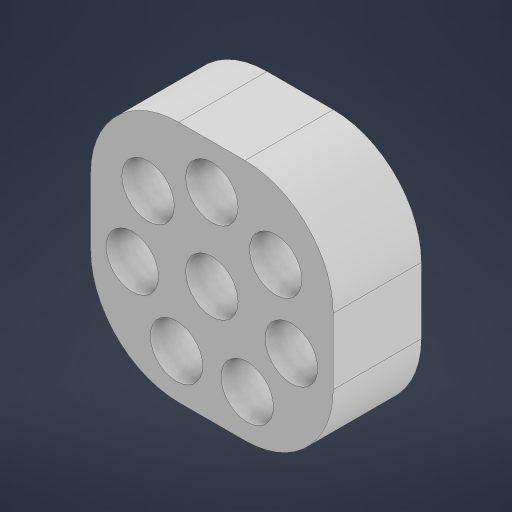
# Autodesk Inventor part: ShooterMount-1in
Saved by Autodesk Inventor 2023 (Build 270158000, 158)
## iProperties
Created: 2022-04-16
Part Number: ShooterMount-1in
Material: Generic
Document SubType Name: Modeling
Designer: timmy
Density: 1 g/cm^3
Appearance: Default
Author: timmy
Autodesk Inventor part; units mm, degrees
ref_plane "YZ Plane" through (0, 0, 0) normal (1, 0, 0) x (0, 1, 0)
sketch "Sketch1" plane through (0, 0, 0) normal (0, 0, 1) x (1, 0, 0)
  line L0 (0, 0) -> (279.4, 0)
  line L1 (279.4, 0) -> (279.4, 279.4)
  line L2 (279.4, 279.4) -> (0, 279.4)
  line L3 (0, 279.4) -> (0, 0)
  circle A0 centre (139.7, 134.62) radius 30.1752
  circle A1 centre (139.7, 228.6) radius 30.1752
  circle A2 centre (66.2235, 193.2156) radius 30.1752
  circle A3 centre (48.0763, 113.7075) radius 30.1752
  circle A4 centre (98.9236, 49.9469) radius 30.1752
  circle A5 centre (180.4764, 49.9469) radius 30.1752
  circle A6 centre (231.3237, 113.7075) radius 30.1752
  circle A7 centre (213.1765, 193.2156) radius 30.1752
  dimension "d0" = 279.4
  dimension "d1" = 279.4
  dimension "d2" = 60.3504
  dimension "d3" = 60.3504
  dimension "d22" = 360
  constraints: 8 centre point, 8 end point, 2 parallel, 1 horizontal, 1 perpendicular, 15 other
  measures "d0" distance of L2.end L1.end
  measures "d1" distance of L1.end L0.end
  measures "d2" diameter of A0
  measures "d3" diameter of A1
extrude "Extrusion1" add sketch "Sketch1" along normal blind 101.6
fillet "Fillet1" radius 101.6 4 edges at (279.4, 279.4, 50.8) (0, 279.4, 50.8) (279.4, 0, 50.8) (0, 0, 50.8)
ref_plane "Work Plane1" through (139.7, 101.6, 0) normal (1, 0, 0) x (0, 0, -1)
ref_plane "Work Plane2" through (0, 0, 50.8) normal (0, 0, 1) x (1, 0, 0)
sketch "Sketch2" plane through (279.4, 101.6, 0) normal (1, 0, 0) x (0, 0, -1)
  line L0 (0, 0) -> (-101.6, 0) projected
  line L1 (0, 0) -> (0, 76.2) projected
  line L2 (-101.6, 76.2) -> (0, 76.2) projected
  line L3 (-101.6, 0) -> (-101.6, 76.2) projected
  circle A0 centre (-50.8, 38.1) radius 12.7
  point P0 (0, -101.6)
  dimension "d14" = 25.4
  constraints: 1 centre point
  measures "d14" diameter of A0
sketch "Sketch3" plane through (0, 101.6, 0) normal (-1, 0, 0) x (0, 0, 1)
  line L0 (101.6, 0) -> (0, 0) projected
  line L1 (101.6, 76.2) -> (101.6, 0) projected
  line L2 (0, 76.2) -> (101.6, 76.2) projected
  line L3 (0, 76.2) -> (0, 0) projected
  circle A0 centre (50.8, 38.1) radius 12.7
  point P0 (0, -101.6)
  dimension "d15" = 25.4
  constraints: 1 centre point
  measures "d15" diameter of A0
body "Solid1"
